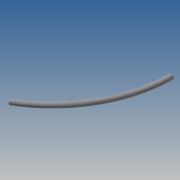
# Autodesk Inventor part: feed-bppvcarc
Saved by Autodesk Inventor 2013 SP2 (Build 170200200, 200)
## iProperties
Created: 2013-07-11
Part Number: feed-bppvcarc
Material: Generic
Document SubType Name: Modeling
Designer: Dave
Density: 1 g/cm^3
Author: Dave
Autodesk Inventor part; units mm, degrees
ref_plane "YZ Plane" through (0, 0, 0) normal (1, 0, 0) x (0, 1, 0)
ref_plane "XZ Plane" through (0, 0, 0) normal (0, 1, 0) x (-1, 0, 0)
ref_plane "XY Plane" through (0, 0, 0) normal (0, 0, 1) x (1, 0, 0)
sketch "Sketch1" plane through (0, 0, 0) normal (0, 0, 1) x (1, 0, 0)
  circle A0 centre (596.9, -0.0117) radius 13.335
  line L0 (0, 80.9625) -> (0, -95.25)
  circle A1 centre (596.9, -0.0117) radius 10.4648
  dimension "d6" = 26.67
  dimension "d7" = 596.9
  dimension "d9" = 2.8702
  constraints: 2 centre point, 2 end point, 1 coincident, 1 vertical
  measures "d6" diameter of A0
  measures "d7" distance from line of L0 A0.centre
  measures "d9" radial gap between concentric circles of A1 A0
revolve "Revolution1" add sketch "Sketch1" angle 60 about axis through (0, 80.9625, 0) along (0, -1, 0)
body "Solid1"
